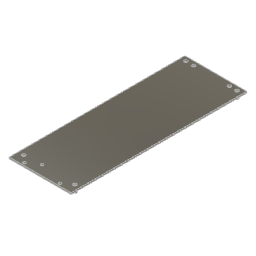
Left Console - Left Aux Spacer v15 (Autodesk Fusion 360 archive; units mm, degrees)
design "Wingwing Base Plate"
Autodesk Fusion 360 part; units mm, degrees
sketch "Sketch1" plane through (0, 0, 0) normal (0, 0, 1) x (1, 0, 0)
  arc A0 (5.4685, 264.659) -> (10.6685, 264.659) centre (8.0685, 264.659) cw
  arc A1 (72.3733, 264.659) -> (77.5733, 264.659) centre (74.9733, 264.659) cw
  arc A2 (89.4019, 264.659) -> (84.2019, 264.659) centre (86.8019, 264.659) cw
  arc A3 (77.5733, 264.659) -> (72.3733, 264.659) centre (74.9733, 264.659) cw
  arc A4 (17.24, 264.659) -> (22.44, 264.659) centre (19.84, 264.659) cw
  arc A5 (10.6685, 264.659) -> (5.4685, 264.659) centre (8.0685, 264.659) cw
  arc A6 (22.44, 264.659) -> (17.24, 264.659) centre (19.84, 264.659) cw
  arc A7 (84.2019, 264.659) -> (89.4019, 264.659) centre (86.8019, 264.659) cw
  arc A8 (11.0257, 13.959) -> (5.8257, 13.959) centre (8.4257, 13.959) cw
  arc A9 (37.7256, 15.1923) -> (33.5256, 15.1923) centre (35.6256, 15.1923) cw
  arc A10 (89.759, 13.959) -> (84.559, 13.959) centre (87.159, 13.959) cw
  arc A11 (17.0257, 4.1923) -> (21.2257, 4.1923) centre (19.1257, 4.1923) cw
  arc A12 (84.559, 13.959) -> (89.759, 13.959) centre (87.159, 13.959) cw
  line L0 (95.3423, 271.0423) -> (0.0423, 271.0423)
  line L1 (95.3423, 0.0423) -> (95.3423, 271.0423)
  arc A13 (33.5256, 15.1923) -> (37.7256, 15.1923) centre (35.6256, 15.1923) cw
  line L2 (0.0423, 271.0423) -> (0.0423, 0.0423)
  arc A14 (21.2257, 4.1923) -> (17.0257, 4.1923) centre (19.1257, 4.1923) cw
  line L3 (0.0423, 0.0423) -> (95.3423, 0.0423)
  arc A15 (76.359, 4.1923) -> (72.159, 4.1923) centre (74.259, 4.1923) cw
  arc A16 (5.8257, 13.959) -> (11.0257, 13.959) centre (8.4257, 13.959) cw
  arc A17 (72.159, 4.1923) -> (76.359, 4.1923) centre (74.259, 4.1923) cw
  circle A18 centre (8.4257, 13.959) radius 2.6
  circle A19 centre (87.159, 13.959) radius 2.6
  constraint concentric A16 A18
  constraint concentric A12 A19
extrude "Extrude1" add sketch "Sketch1" along normal blind 2.2 makes body 1
extrude "Extrude2" add sketch "Sketch1" against normal blind 7.8 separate body contours A0 A5 | A2 A7 | A8 A16 A18 | A10 A12 A19 makes body 2 at (87.4823, 16.5388, -5.2) makes body 3 at (10.4644, 265.6689, -2.6) makes body 4 at (5.8386, 14.2179, -5.2) makes body 5 at (89.2451, 263.7697, -2.6)
